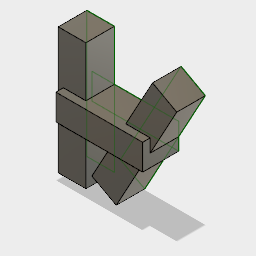
TwentyOnePilots-logo v1 (Autodesk Fusion 360 design; units mm, degrees)
Autodesk Fusion 360 part; units mm, degrees
sketch "Sketch1" plane through (0, 0, 0) normal (0, 0, 1) x (1, 0, 0)
  line L0 (-41.2185, 94.5561) -> (-4.3961, 94.5561)
  line L1 (-4.3961, 94.5561) -> (-4.3961, -73.6817)
  line L2 (-4.3961, -73.6817) -> (-41.2185, -73.6817)
  line L3 (-41.2185, -73.6817) -> (-41.2185, 94.5561)
  line L4 (84.0952, 92.7118) -> (116.424, 75.0841)
  line L5 (116.424, 75.0841) -> (35.8844, -72.6229)
  line L6 (35.8844, -72.6229) -> (3.5557, -54.9951)
  line L7 (3.5557, -54.9951) -> (84.0952, 92.7118)
  line L8 (81.0854, 27.7563) -> (81.0854, -6.6095)
  line L9 (81.0854, -6.6095) -> (-34.3246, -6.6095)
  line L10 (-34.3246, -6.6095) -> (-34.3246, 27.7563)
  line L11 (-34.3246, 27.7563) -> (81.0854, 27.7563)
extrude "Extrude2" add sketch "Sketch1" along normal blind 48 contours L1 L7 L9 L11 | L1 L9 L10 L11 | L5 L7 L8 L9 L11 | L5 L8 L9 makes body 1
extrude "Extrude1" add sketch "Sketch1" along normal blind 38 separate body contours L0 L1 L2 L3 L9 L10 L11 makes body 2
extrude "Extrude3" add sketch "Sketch1" along normal blind 38 separate body contours L5 L6 L7 L9 makes body 3
extrude "Extrude4" add sketch "Sketch1" along normal blind 38 separate body contours L4 L5 L7 L8 L11 makes body 4
combine "Combine1" operation add target body 4 tool bodies 3 2 1
named bodies: "First", "Middle", "SecondBottom", "TopLogo"
